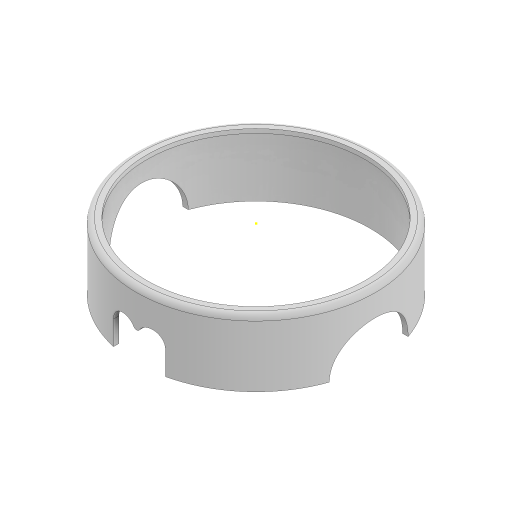
# Autodesk Inventor part: Shell-disc
Saved by Autodesk Inventor 2024 (Build 280153000, 153)
## iProperties
Created: 2025-10-21
Part Number: Shell-disc
Material: 一般
Document SubType Name: Modeling
Designer: USER
Density: 1 g/cm^3
Appearance: 預設
Author: USER
Autodesk Inventor part; units mm, degrees
ref_plane "YZ Plane" through (0, 0, 0) normal (1, 0, 0) x (0, 1, 0)
ref_plane "XZ Plane" through (0, 0, 0) normal (0, 1, 0) x (-1, 0, 0)
ref_plane "XY Plane" through (0, 0, 0) normal (0, 0, 1) x (1, 0, 0)
sketch "草圖1" plane through (0, 0, 0) normal (0, 1, 0) x (-1, 0, 0)
  circle A0 centre (0, 0) radius 110
  dimension "d0" = 220
  constraints: 1 centre point, 1 coincident
  measures "d0" diameter of A0
extrude "擠出1" add sketch "草圖1" along normal blind 4
sketch "草圖2" plane through (0, 4, 0) normal (0, 1, 0) x (1, 0, 0)
  circle A0 centre (0, 0) radius 110 projected
sketch "草圖3" plane through (0, 4, 0) normal (0, 1, 0) x (1, 0, 0)
  circle A0 centre (0, 0) radius 110 projected
  circle A1 centre (0, 0) radius 115
  circle A2 centre (0, 0) radius 105
  dimension "d3" = 5
  dimension "d4" = 5
  constraints: 2 centre point
  measures "d3" radial gap between concentric circles of A0 A1
  measures "d4" radial gap between concentric circles of A0 A2
extrude "擠出2" add sketch "草圖3" against normal blind 59 contours A1
sketch "草圖4" plane through (0, 4, 0) normal (0, 1, 0) x (1, 0, 0)
  circle A0 centre (0, 0) radius 115 projected
  circle A1 centre (0, 0) radius 110
  circle A2 centre (0, 0) radius 105
  dimension "d7" = 5
  constraints: 2 centre point, 1 coincident
  measures "d7" radial gap between concentric circles of A1 A2
extrude "擠出3" add sketch "草圖4" along normal blind 5 contours A0 | A1
sketch "草圖5" plane through (0, 0, 0) normal (0, -1, 0) x (1, 0, 0)
  circle A0 centre (0, 0) radius 110 projected
  circle A1 centre (0, 0) radius 110
  dimension "d10" = 220
  constraints: 1 centre point, 1 coincident
  measures "d10" diameter of A1
extrude "擠出4" cut sketch "草圖5" against normal blind 5
fillet "圓角2" radius 5 1 edges at (-115, 9, 0)
sketch "草圖6" plane through (0, 0, 0) normal (0, 0, 1) x (1, 0, 0)
  line L0 (-115, -55) -> (115, -55) projected
  line L1 (0, -53) -> (25, -53)
  line L2 (0, -53) -> (-25, -53)
  line L3 (-25, -53) -> (-25, -32)
  line L4 (25, -53) -> (25, -32)
  line L5 (-25, -32) -> (-13, -32)
  circle A0 centre (-13, -32) radius 8.1
  arc A1 (-2.7801, -25.7108) -> (-25, -32) centre (-13, -32) ccw
  circle A2 centre (13, -32) radius 8.1
  arc A3 (25, -32) -> (2.7801, -25.7108) centre (13, -32) ccw
  arc A4 (-2.7801, -25.7108) -> (2.7801, -25.7108) centre (0, -24) ccw
  line L6 (0, -55) -> (-25, -55)
  line L7 (-25, -55) -> (-25, -53)
  line L8 (0, -55) -> (25, -55)
  line L9 (25, -53) -> (25, -55)
  point P0 (0, 0)
  dimension "d15" = 25
  dimension "d16" = 25
  dimension "d17" = 21
  dimension "d18" = 21
  dimension "d19" = 12
  dimension "d20" = 16.2
  dimension "d22" = 25
  dimension "d23" = 2
  constraints: 18 end point, 6 point on circle, 5 centre point, 3 coincident, 2 perpendicular, 2 point on line, 2 vertical, 1 horizontal, 1 midpoint, 1 tangent
  measures "d15" distance of L1.start L1.end
  measures "d16" distance of L1.start L2.end
  measures "d17" distance of L2.end L3.end
  measures "d18" distance of L1.end L4.end
  measures "d19" distance of L3.end L5.end
  measures "d20" diameter of A0
  measures "d22" distance of L6.start L6.end
  measures "d23" distance of L6.end L7.end
extrude "擠出5" cut sketch "草圖6" along normal blind 200 contours L7 L2 L1 L9 L0 | A0 | L3 A1 A4 A3 L4 L1 L2 | A2
sketch "草圖7" plane through (0, 0, 0) normal (1, 0, 0) x (0, 1, 0)
  line L0 (-55, 112.2497) -> (-55, -115) projected
  line L1 (-55, 0) -> (-55, -38)
  line L2 (-55, 0) -> (-55, 38)
  circle A0 centre (-55, 0) radius 38
  point P0 (0, 0)
  dimension "d26" = 38
  dimension "d27" = 38
  constraints: 4 end point, 3 point on line, 1 coincident, 3 other
  measures "d26" distance of L1.start L1.end
  measures "d27" distance of L1.start L2.end
extrude "擠出6" cut sketch "草圖7" along normal mid plane 400 contours A0 L0 picked at (-29.9842, -2.8186)
